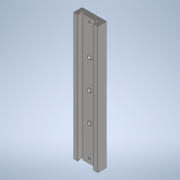
# Autodesk Inventor part: uchwyt_szyny
Saved by Autodesk Inventor 2020 (Build 240168000, 168)
## iProperties
Created: 2020-08-26
Part Number: uchwyt_szyny
Material: Stainless Steel
Document SubType Name: Modeling
Designer: Hesekiel
Density: 8 g/cm^3
Appearance: Semi-Polished
Author: Hesekiel
Autodesk Inventor part; units mm, degrees
ref_plane "YZ Plane" through (0, 0, 0) normal (1, 0, 0) x (0, 1, 0)
ref_plane "XZ Plane" through (0, 0, 0) normal (0, 1, 0) x (-1, 0, 0)
ref_plane "XY Plane" through (0, 0, 0) normal (0, 0, 1) x (1, 0, 0)
sketch "Sketch1" plane through (0, 0, 0) normal (0, 1, 0) x (-1, 0, 0)
  line L0 (37, 0) -> (0, 0)
  line L1 (0, 0) -> (-3.25, -15)
  line L2 (-3.25, -15) -> (3.25, -15)
  line L3 (3.25, -15) -> (3.25, -8.5)
  line L4 (3.25, -8.5) -> (33.75, -8.5)
  line L5 (33.75, -8.5) -> (33.75, -15)
  line L6 (33.75, -15) -> (40.25, -15)
  line L7 (40.25, -15) -> (37, 0)
  line L8 (37, 0) -> (47, 0)
  line L9 (47, 0) -> (47, -20)
  line L10 (47, -20) -> (-10, -20)
  line L11 (-10, -20) -> (-10, 0)
  line L12 (-10, 0) -> (0, 0)
  dimension "d1" = 20
  dimension "d5" = 10
  dimension "d6" = 10
  constraints: 26 end point, 4 perpendicular, 1 horizontal, 1 point on line
  measures "d1" distance of L8.end L9.end
  measures "d5" distance of L11.end point (0, 0)
  measures "d6" distance of L0.start L8.end
extrude "Extrusion1" add sketch "Sketch1" along normal blind 300 contours L8 L9 L10 L11 L12 L1 L2 L3 L4 L5 L6 L7
sketch "Sketch2" plane through (10, 0, -20) normal (0, 0, -1) x (-1, 0, 0)
  line L0 (0, 0) -> (57, 0) projected
  line L1 (57, 0) -> (57, 300) projected
  line L2 (0, 300) -> (57, 300) projected
  line L3 (0, 0) -> (0, 300) projected
  line L4 (43.75, 0) -> (13.25, 0) projected
  line L5 (28.5, 0) -> (28.5, 300)
  line L6 (43.75, 300) -> (13.25, 300) projected
  line L7 (0, 52.5) -> (57, 52.5)
  line L8 (57, 52.5) -> (57, 247.5)
  line L9 (57, 247.5) -> (0, 247.5)
  line L10 (0, 247.5) -> (0, 52.5)
  line L11 (0, 52.5) -> (57, 247.5) construction
  line L12 (57, 52.5) -> (0, 247.5) construction
  circle A0 centre (28.5, 150) radius 3.1
  line L13 (28.5, 52.5) -> (28.5, 82.5)
  circle A1 centre (28.5, 82.5) radius 3.1
  line L14 (28.5, 247.5) -> (28.5, 217.5)
  circle A2 centre (28.5, 217.5) radius 3.1
  point P0 (10, 0)
  dimension "d7" = 195
  dimension "d8" = 6.2
  dimension "d9" = 30
  dimension "d10" = 6.2
  dimension "d11" = 30
  dimension "d12" = 6.2
  constraints: 18 end point, 7 midpoint, 3 centre point, 3 coincident, 3 point on line, 2 parallel, 1 horizontal, 1 perpendicular
  measures "d7" distance of L8.end L7.end
  measures "d8" diameter of A0
  measures "d9" distance of L13.start L13.end
  measures "d10" diameter of A1
  measures "d11" distance of L14.start L14.end
  measures "d12" diameter of A2
extrude "Extrusion2" cut sketch "Sketch2" against normal up to surface (11.5 mm away) contours A1 L5 | L5 A1 | A2 L5 | L5 A2 | A0 L5 | L5 A0
sketch "Sketch4" plane through (-33.75, 0, -8.5) normal (0, 0, 1) x (1, 0, 0)
  circle A0 centre (15.25, 217.5) radius 3.1 projected
  circle A1 centre (15.25, 82.5) radius 3.1 projected
  circle A2 centre (15.25, 150) radius 3.1 projected
  line L0 (0, 0) -> (30.5, 0) projected
  line L1 (30.5, 0) -> (30.5, 300) projected
  line L2 (0, 300) -> (30.5, 300) projected
  line L3 (0, 0) -> (0, 300) projected
  circle A3 centre (15.25, 82.5) radius 3.1 projected
  circle A4 centre (15.25, 82.5) radius 5
  circle A5 centre (15.25, 150) radius 5
  circle A6 centre (15.25, 217.5) radius 5
  point P0 (33.75, 0)
  dimension "d15" = 10
  dimension "d16" = 10
  dimension "d17" = 10
  constraints: 3 centre point, 3 coincident
  measures "d15" diameter of A4
  measures "d16" diameter of A5
  measures "d17" diameter of A6
extrude "Extrusion3" cut sketch "Sketch4" against normal blind 6 contours A4 | A5 | A6
sketch "Sketch5" plane through (-33.75, 0, -8.5) normal (0, 0, 1) x (1, 0, 0)
  line L0 (43.75, 0) -> (-13.25, 0) projected
  line L1 (15.25, 0) -> (15.25, 10)
  line L2 (43.75, 300) -> (-13.25, 300) projected
  line L3 (15.25, 300) -> (15.25, 290)
  circle A0 centre (15.25, 290) radius 2.5
  circle A1 centre (15.25, 10) radius 2.5
  point P0 (33.75, 0)
  dimension "d20" = 10
  dimension "d21" = 10
  dimension "d22" = 5
  dimension "d23" = 5
  constraints: 4 end point, 2 centre point, 2 coincident, 2 midpoint, 2 vertical
  measures "d20" distance of L1.start L1.end
  measures "d21" distance of L3.start L3.end
  measures "d22" diameter of A0
  measures "d23" diameter of A1
extrude "Extrusion4" cut sketch "Sketch5" against normal up to surface (11.5 mm away)
thread "Thread1" size "M5x0.8" class "6H" standard "ANSI Metric M Profile" full length
thread "Thread2" size "M5x0.8" class "6H" standard "ANSI Metric M Profile" full length
body "Solid1"
